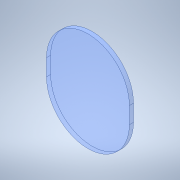
# Autodesk Inventor part: 20_cube_circular_polarizer
Saved by Autodesk Inventor 2022 (Build 260153000, 153)
## iProperties
Created: 2020-10-09
Part Number: 20_cube_circular_polarizer
Material: Generisch
Document SubType Name: Blech
Designer: UC2
Density: 1 g/cm^3
Sheet Metal Rule: Default
Appearance: Vorgabe
Author: UC2
Autodesk Inventor part; units mm, degrees
ref_plane "YZ Plane" through (0, 0, 0) normal (1, 0, 0) x (0, 1, 0)
ref_plane "XZ Plane" through (0, 0, 0) normal (0, 1, 0) x (-1, 0, 0)
ref_plane "XY Plane" through (0, 0, 0) normal (0, 0, 1) x (1, 0, 0)
sketch "Skizze1" plane through (0, 0, 0) normal (0, 0, 1) x (1, 0, 0)
  line L0 (0, 19.9048) -> (0, -28.0952) construction
  line L1 (-20, -0.0952) -> (-20, -8.0952)
  line L2 (20, -8.0952) -> (20, -0.0952)
  arc A0 (20, -0.0952) -> (-20, -0.0952) centre (0, -0.0952) ccw
  arc A1 (-20, -8.0952) -> (20, -8.0952) centre (0, -8.0952) ccw
  point P0 (0, 0)
  point P1 (0, -4.0952)
  dimension "d0" = 40
  dimension "d1" = 48
  constraints: 8 end point, 6 point on circle, 4 tangent, 2 centre point, 2 point on line, 1 midpoint, 1 parallel, 1 vertical
  measures "d0" distance between parallel lines of L2 L1
  measures "d1" distance of L0.end L0.start
extrude "Extrusion1" add sketch "Skizze1" along normal blind 2
equation "\"Biegeradius\" = Stärke"
equation "\"BreiteBiegungsfreistellung\" = Stärke"
equation "\"TiefeBiegungsfreistellung\" = 0.5 * Stärke"
equation "\"GrößeEckenfreistellung\" = 4 * Stärke"
equation "\"MinimalRest\" = 2 * Stärke"
equation "\"Übergangsradius\" = Biegeradius"
equation "\"JacobiRadiusGröße\" = Biegeradius"
equation "\"Abstandsgröße\" = Stärke"
equation "\"Stärke\" = 3.048"
